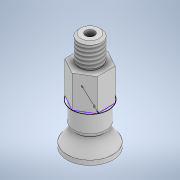
# Autodesk Inventor part: cup
Saved by Autodesk Inventor 2021 (Build 250183000, 183)
## iProperties
Created: 2020-11-29
Part Number: cup
Material: Generic
Document SubType Name: Modeling
Designer: awitc
Density: 1 g/cm^3
Appearance: Default
Author: awitc
Autodesk Inventor part; units mm, degrees
ref_plane "YZ Plane" through (0, 0, 0) normal (1, 0, 0) x (0, 1, 0)
ref_plane "XZ Plane" through (0, 0, 0) normal (0, 1, 0) x (-1, 0, 0)
ref_plane "XY Plane" through (0, 0, 0) normal (0, 0, 1) x (1, 0, 0)
sketch "Sketch1" plane through (0, 0, 0) normal (0, 1, 0) x (-1, 0, 0)
  circle A0 centre (0, 0) radius 5
  circle A1 centre (0, 0) radius 3
  dimension "d35" = 10
  dimension "d36" = 6
  constraints: 2 centre point, 1 coincident
  measures "d35" diameter of A0
  measures "d36" diameter of A1
extrude "Extrusion11" add sketch "Sketch1" along normal blind 4 contours A1
extrude "Extrusion12" add sketch "Sketch1" along normal blind 1
draft "FaceDraft2" angle 33.5 pull direction (0, 1, 0) faces at (-2.9903, 3, -0.2414) fixed edges at (3, 4, 0)
sketch "Sketch8" plane through (0, 4, 0) normal (0, 1, 0) x (1, 0, 0)
  circle A0 centre (0, 0) radius 3.5
  dimension "d42" = 7
  constraints: 1 centre point, 1 coincident
  measures "d42" diameter of A0
extrude "Extrusion13" add sketch "Sketch8" along normal blind 5
chamfer "Chamfer2" distance 0.5 angle 45 1 edges at (-3.5, 4, 0)
fillet "Fillet1" radius 1 1 edges at (-3.5, 4.4999, 0)
sketch "Sketch9" plane through (0, 9, 0) normal (0, 1, 0) x (1, 0, 0)
  circle A0 centre (0, 0) radius 4
  line L0 (3.5, -1.9365) -> (0.0729, -3.9993)
  line L1 (0.0729, -3.9993) -> (-3.4271, -2.0628)
  line L2 (-3.4271, -2.0628) -> (-3.5, 1.9365)
  line L3 (-3.5, 1.9365) -> (-0.0729, 3.9993)
  line L4 (-0.0729, 3.9993) -> (3.4271, 2.0628)
  line L5 (3.4271, 2.0628) -> (3.5, -1.9365)
  circle A1 centre (0, 0) radius 3.5
  point P0 (1.3581, -3.2258)
  point P1 (-1.2396, -3.2732)
  point P2 (-2.1146, -2.789)
  point P3 (-3.4544, -0.5631)
  point P4 (-3.4726, 0.4367)
  point P5 (-2.2149, 2.7101)
  point P6 (-1.3581, 3.2258)
  point P7 (1.2396, 3.2732)
  point P8 (2.1146, 2.789)
  point P9 (3.4544, 0.5631)
  point P10 (3.4726, -0.4367)
  point P11 (2.2149, -2.7101)
  dimension "d49" = 8
  constraints: 12 end point, 3 coincident, 1 centre point, 16 other
extrude "Extrusion14" add sketch "Sketch9" along normal blind 7 contours L5 A1 L4 | L0 A1 L5 | L4 A1 L3 | A1 L5 L0 L1 L2 L3 L4 | L1 A1 L0 | L3 A1 L2 | L2 A1 L1
sketch "Sketch10" plane through (0, 16, 0) normal (0, 1, 0) x (1, 0, 0)
  circle A0 centre (0, 0) radius 2.5
  circle A1 centre (0, 0) radius 2.25
  dimension "d54" = 5
  dimension "d55" = 4.5
  constraints: 2 centre point, 2 coincident
  measures "d54" diameter of A0
  measures "d55" diameter of A1
extrude "Extrusion16" add sketch "Sketch10" along normal blind 0.5 contours A1
sketch "Sketch11" plane through (0, 16.5, 0) normal (0, 1, 0) x (1, 0, 0)
  circle A0 centre (0, 0) radius 2.5
  dimension "d58" = 5
  constraints: 1 centre point, 1 coincident
  measures "d58" diameter of A0
extrude "Extrusion18" add sketch "Sketch11" along normal blind 5
fillet "Fillet2" radius 0.5 1 edges at (-2.25, 16.5, 0)
thread "Thread2" size "M5x0.8" class "6g" standard "ANSI Metric M Profile" full length
chamfer "Chamfer3" distance 0.5 angle 45 1 edges at (-2.5, 21.5, 0)
sketch "Sketch12" plane through (0, 0, 0) normal (0, -1, 0) x (1, 0, 0)
  circle A0 centre (0, 0) radius 4
  dimension "d70" = 8
  constraints: 1 centre point, 1 coincident
  measures "d70" diameter of A0
extrude "Extrusion19" cut sketch "Sketch12" against normal blind 2
fillet "Fillet3" radius 0.5 1 edges at (-4, 2, 0)
sketch "Sketch13" plane through (0, 21.5, 0) normal (0, 1, 0) x (1, 0, 0)
  circle A0 centre (0, 0) radius 1
  dimension "d74" = 2
  constraints: 1 centre point, 1 coincident
  measures "d74" diameter of A0
extrude "Extrusion20" cut sketch "Sketch13" against normal up to next
body "Solid2"
